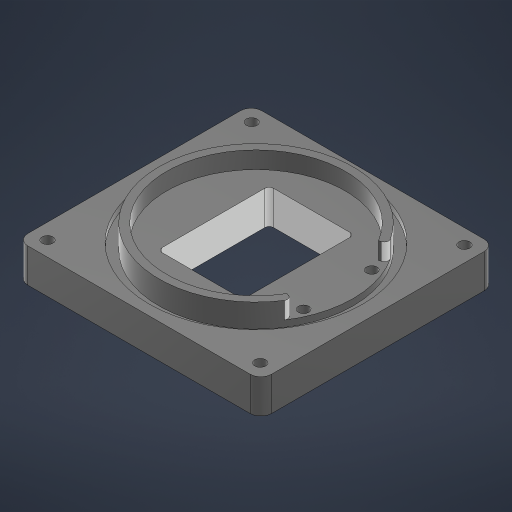
# Autodesk Inventor part: UnitV_Mount
Saved by Autodesk Inventor 2024.2 (Build 282272000, 272)
## iProperties
Created: 2024-02-19
Part Number: UnitV_Mount
Material: 一般
Document SubType Name: Modeling
Designer: Hanaoka
Density: 1 g/cm^3
Appearance: 既定
Author: Hanaoka
Autodesk Inventor part; units mm, degrees
ref_plane "YZ Plane" through (0, 0, 0) normal (1, 0, 0) x (0, 1, 0)
ref_plane "XZ Plane" through (0, 0, 0) normal (0, 1, 0) x (-1, 0, 0)
ref_plane "XY Plane" through (0, 0, 0) normal (0, 0, 1) x (1, 0, 0)
sketch "スケッチ1" plane through (0, 0, 0) normal (0, 1, 0) x (-1, 0, 0)
  line L0 (-25, 24) -> (25, 24) construction
  line L1 (25, 24) -> (25, -24) construction
  line L2 (25, -24) -> (-25, -24) construction
  line L3 (-25, -24) -> (-25, 24) construction
  line L4 (-25, 24) -> (25, -24) construction
  line L5 (25, 24) -> (-25, -24) construction
  line L6 (-26.1458, 27.5) -> (26.1458, 27.5)
  line L7 (28.6458, 25) -> (28.6458, -25)
  line L8 (26.1458, -27.5) -> (-26.1458, -27.5)
  line L9 (-28.6458, -25) -> (-28.6458, 25)
  line L10 (-28.6458, 27.5) -> (28.6458, -27.5) construction
  line L11 (28.6458, 27.5) -> (-28.6458, -27.5) construction
  arc A0 (28.6458, 25) -> (26.1458, 27.5) centre (26.1458, 25) ccw
  arc A1 (26.1458, -27.5) -> (28.6458, -25) centre (26.1458, -25) ccw
  arc A2 (-28.6458, -25) -> (-26.1458, -27.5) centre (-26.1458, -25) ccw
  arc A3 (-26.1458, 27.5) -> (-28.6458, 25) centre (-26.1458, 25) ccw
  circle A4 centre (25, 24) radius 1.3
  circle A5 centre (25, -24) radius 1.3
  circle A6 centre (-25, 24) radius 1.3
  circle A7 centre (-25, -24) radius 1.3
  point P0 (0, 0)
  dimension "d0" = 50
  dimension "d1" = 48
  dimension "d2" = 2.5
  dimension "d3" = 2.6
  dimension "d4" = 50
  constraints: 24 end point, 12 point on line, 8 centre point, 8 point on circle, 8 tangent, 6 equal radius, 4 midpoint, 4 parallel, 2 horizontal, 2 perpendicular, 1 coincident
  measures "d0" distance of L0.start L0.end
  measures "d1" distance of L1.end L0.end
  measures "d2" radius of A0
  measures "d3" diameter of A6
  measures "d4" distance of L7.start L7.end
extrude "押し出し1" add sketch "スケッチ1" along normal blind 8
sketch "スケッチ2" plane through (0, 8, 0) normal (0, 1, 0) x (1, 0, 0)
  circle A0 centre (0, 0) radius 22.825
  line L0 (26.1458, 27.5) -> (-26.1458, 27.5) projected
  arc A1 (-26.1458, 27.5) -> (-28.6458, 25) centre (-26.1458, 25) ccw projected
  line L1 (-28.6458, 25) -> (-28.6458, -25) projected
  arc A2 (-28.6458, -25) -> (-26.1458, -27.5) centre (-26.1458, -25) ccw projected
  line L2 (-26.1458, -27.5) -> (26.1458, -27.5) projected
  arc A3 (26.1458, -27.5) -> (28.6458, -25) centre (26.1458, -25) ccw projected
  line L3 (28.6458, -25) -> (28.6458, 25) projected
  arc A4 (28.6458, 25) -> (26.1458, 27.5) centre (26.1458, 25) ccw projected
  circle A5 centre (25, 24) radius 1.3 projected
  circle A6 centre (25, -24) radius 1.3 projected
  circle A7 centre (-25, 24) radius 1.3 projected
  circle A8 centre (-25, -24) radius 1.3 projected
  circle A9 centre (0, 0) radius 25.1
  circle A10 centre (0, 0) radius 21
  dimension "d7" = 45.65
  dimension "d9" = 50.2
  dimension "d10" = 42
  constraints: 3 centre point, 2 coincident
  measures "d7" diameter of A0
  measures "d9" diameter of A9
  measures "d10" diameter of A10
extrude "押し出し2" cut sketch "スケッチ2" against normal blind 1.5 contours A9
extrude "押し出し6" add sketch "スケッチ2" along normal blind 4 contours A0
sketch "スケッチ5" plane through (0, 8, 0) normal (0, 1, 0) x (1, 0, 0)
  line L0 (9, -12.1) -> (-9, -12.1)
  line L1 (-9, -12.1) -> (-9, 12.1)
  line L2 (-9, 12.1) -> (9, 12.1)
  line L3 (9, 12.1) -> (9, -12.1)
  line L4 (9, -12.1) -> (-9, 12.1) construction
  line L5 (-9, -12.1) -> (9, 12.1) construction
  circle A0 centre (19.2, -8) radius 1.25
  circle A1 centre (19.2, 8) radius 1.25
  line L6 (31, 12) -> (-9, 12) construction
  line L7 (-9, -12) -> (31, -12) construction
  line L8 (31, -12) -> (31, 12) construction
  line L9 (31, 12) -> (-9, -12) construction
  line L10 (-9, 12) -> (31, -12) construction
  line L11 (0, 0) -> (28.6458, 0) construction
  line L12 (28.6458, -25) -> (28.6458, 25) projected
  line L13 (19.2, -8) -> (19.2, 8) construction
  circle A2 centre (19.2, -8) radius 3
  circle A3 centre (19.2, 8) radius 3
  circle A4 centre (0, 0) radius 22.825 projected
  circle A5 centre (0, 0) radius 21 projected
  point P0 (11, 0)
  point P1 (20.3396, -5.2249)
  point P2 (21.8512, -6.596)
  point P3 (21.8512, 6.596)
  point P4 (20.3396, 5.2249)
  dimension "d33" = 18
  dimension "d34" = 24.2
  dimension "d35" = 2.5
  dimension "d37" = 24
  dimension "d38" = 40
  dimension "d39" = 11.8
  dimension "d40" = 16
  dimension "d41" = 6
  constraints: 26 end point, 5 midpoint, 4 centre point, 3 parallel, 2 coincident, 2 equal radius, 2 horizontal, 1 perpendicular, 1 point on line, 1 vertical, 2 other
  measures "d33" distance of L1.end L2.end
  measures "d34" distance of L0.end L1.end
  measures "d35" diameter of A0
  measures "d37" distance of L7.end L6.start
  measures "d38" distance of L6.start L6.end
  measures "d39" distance between parallel lines of L8 L13
  measures "d40" distance of L13.start L13.end
  measures "d41" diameter of A2
extrude "押し出し7" cut sketch "スケッチ5" along normal blind 4 contours A0 A5 | A0 A5 A2 A4 | A5 A0 | A0 A5 A2 | A5 A3 A4 A2 | A2 A4 | A5 A1 A3 | A3 A4 A5 A1 | A3 A4 | A5 A1 | A1 A5 picked at (22.1558, -1.3283)
extrude "押し出し8" cut sketch "スケッチ5" against normal up to surface (8 mm away) contours L0 L1 L2 L3 | A0 A5 | A5 A0 | A5 A1 | A1 A5
sketch "スケッチ6" plane through (0, 8, 0) normal (0, 1, 0) x (1, 0, 0)
  circle A0 centre (19.2, 8) radius 1.25 projected
  line L0 (-9, 12.1) -> (9, 12.1) projected
  line L1 (9, 12.1) -> (9, -12.1) projected
  line L2 (9, -12.1) -> (-9, -12.1) projected
  line L3 (-9, -12.1) -> (-9, 12.1) projected
  circle A1 centre (19.2, -8) radius 1.25 projected
  arc A2 (18.032, -10.7633) -> (20.0699, -10.8711) centre (19.2, -8) ccw projected
  arc A3 (20.0699, -10.8711) -> (20.0699, 10.8711) centre (0, 0) ccw projected
  arc A4 (20.0699, 10.8711) -> (18.032, 10.7633) centre (19.2, 8) ccw projected
  arc A5 (18.032, 10.7633) -> (18.032, -10.7633) centre (0, 0) ccw projected
  line L4 (10, -13.1) -> (-10, -13.1)
  line L5 (-10, -13.1) -> (-10, 13.1)
  line L6 (-10, 13.1) -> (10, 13.1)
  line L7 (10, 13.1) -> (10, -13.1)
  line L8 (10, -13.1) -> (-10, 13.1) construction
  line L9 (-10, -13.1) -> (10, 13.1) construction
  dimension "d46" = 1
  dimension "d47" = 1
  constraints: 12 end point, 2 midpoint, 2 parallel, 1 horizontal, 1 perpendicular
  measures "d46" distance between parallel lines of L4 L2
  measures "d47" distance between parallel lines of L3 L5
extrude "押し出し9" cut sketch "スケッチ6" against normal up to surface (8 mm away) contours L4 L5 L6 L7
fillet "フィレット1" radius 1 6 edges at (-10, 4, 13.1) (10, 4, 13.1) (10, 4, -13.1) (-10, 4, -13.1) (20.0699, 10, 10.8711) (20.0699, 10, -10.8711)
sketch "スケッチ7" plane through (0, 0, 0) normal (0, -1, 0) x (1, 0, 0)
  line L0 (9, -13.1) -> (-9, -13.1) projected
  arc A0 (-10, -12.1) -> (-9, -13.1) centre (-9, -12.1) ccw projected
  line L1 (-10, -12.1) -> (-10, 12.1) projected
  arc A1 (-9, 13.1) -> (-10, 12.1) centre (-9, 12.1) ccw projected
  line L2 (-9, 13.1) -> (9, 13.1) projected
  arc A2 (10, 12.1) -> (9, 13.1) centre (9, 12.1) ccw projected
  line L3 (10, 12.1) -> (10, -12.1) projected
  arc A3 (9, -13.1) -> (10, -12.1) centre (9, -12.1) ccw projected
  circle A4 centre (19.2, -8) radius 1.25 projected
  circle A5 centre (19.2, 8) radius 1.25 projected
  line L4 (26.1458, -27.5) -> (-26.1458, -27.5) projected
  arc A6 (26.1458, -27.5) -> (28.6458, -25) centre (26.1458, -25) ccw projected
  line L5 (28.6458, 25) -> (28.6458, -25) projected
  arc A7 (28.6458, 25) -> (26.1458, 27.5) centre (26.1458, 25) ccw projected
  line L6 (-26.1458, 27.5) -> (26.1458, 27.5) projected
  arc A8 (-26.1458, 27.5) -> (-28.6458, 25) centre (-26.1458, 25) ccw projected
  line L7 (-28.6458, -25) -> (-28.6458, 25) projected
  arc A9 (-28.6458, -25) -> (-26.1458, -27.5) centre (-26.1458, -25) ccw projected
  circle A10 centre (25, -24) radius 1.3 projected
  circle A11 centre (25, 24) radius 1.3 projected
  circle A12 centre (-25, -24) radius 1.3 projected
  circle A13 centre (-25, 24) radius 1.3 projected
  line L8 (9, -13.1) -> (23, -13.1)
  line L9 (23, -13.1) -> (23, 13.1)
  line L10 (23, 13.1) -> (9, 13.1)
  line L11 (10, 12.1) -> (10, -12.1) projected
  point P0 (0, 0)
  dimension "d52" = 14
  constraints: 6 end point, 2 parallel, 1 horizontal
  measures "d52" distance of L0.start L8.end
extrude "押し出し10" add sketch "スケッチ7" along normal blind 1.5 contours A3 L3 A2 L10 L9 L8
equation "\"d47\" = d46"
